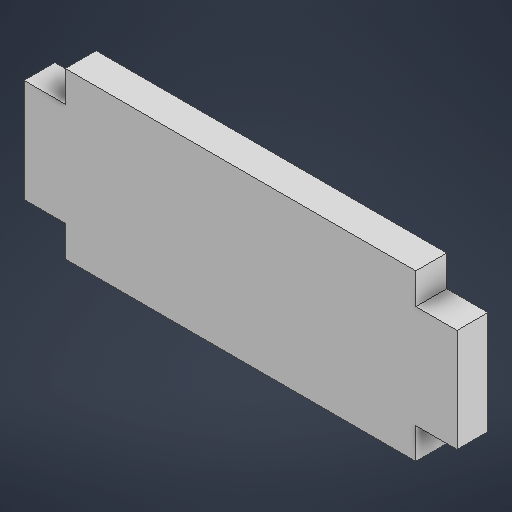
# Autodesk Inventor part: Frontrail
Saved by Autodesk Inventor 2027 (Build 310192000, 192)
## iProperties
Created: 2026-05-13
Part Number: Frontrail
Material: Generic
Document SubType Name: Modeling
Designer: alexy
Density: 1 g/cm^3
Appearance: Default
Author: alexy
Autodesk Inventor part; units mm, degrees
ref_plane "YZ Plane" through (0, 0, 0) normal (1, 0, 0) x (0, 1, 0)
ref_plane "XZ Plane" through (0, 0, 0) normal (0, 1, 0) x (-1, 0, 0)
ref_plane "XY Plane" through (0, 0, 0) normal (0, 0, 1) x (1, 0, 0)
sketch "Sketch1" plane through (0, 0, 0) normal (0, 0, 1) x (1, 0, 0)
  line L0 (0, 0) -> (34, 0)
  line L1 (34, 0) -> (34, 16)
  line L2 (34, 16) -> (0, 16)
  line L3 (0, 16) -> (0, 0)
  line L4 (-4, 13) -> (0, 13)
  line L5 (0, 13) -> (0, 3)
  line L6 (0, 3) -> (-4, 3)
  line L7 (-4, 3) -> (-4, 13)
  line L8 (-4, 13) -> (0, 3) construction
  line L9 (0, 13) -> (-4, 3) construction
  line L10 (38, 13) -> (34, 13)
  line L11 (34, 13) -> (34, 3)
  line L12 (34, 3) -> (38, 3)
  line L13 (38, 3) -> (38, 13)
  line L14 (38, 13) -> (34, 3) construction
  line L15 (34, 13) -> (38, 3) construction
  point P0 (-2, 8)
  point P1 (36, 8)
  point P2 (0, 8)
  point P3 (0, 8)
  point P4 (0, 13)
  dimension "d0" = 34
  dimension "d1" = 16
  dimension "d2" = 4
  dimension "d3" = 4
  dimension "d4" = 10
  dimension "d5" = 10
  constraints: 32 end point, 6 midpoint, 6 parallel, 3 horizontal, 3 perpendicular, 2 horizontal alignment, 2 point on line
  measures "d0" distance of L1.end L2.end
  measures "d1" distance of L0.end L1.end
  measures "d2" distance of L10.start L10.end
  measures "d3" distance of L4.start L4.end
  measures "d4" distance of L6.end L4.start
  measures "d5" distance of L12.end L10.start
extrude "Extrusion1" add sketch "Sketch1" along normal blind 3
body "Solid1"
